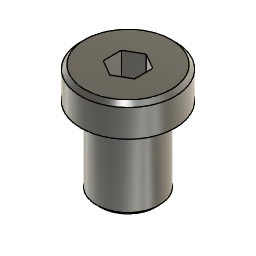
Ensamble+Piezas+SW (Autodesk Fusion 360 archive; units mm, degrees)
design "Cuarta Pieza SW"
Autodesk Fusion 360 part; units mm, degrees
sketch "Sketch1" plane through (0, 0, 0) normal (0, 0, 1) x (1, 0, 0)
  circle A0 centre (0, 0) radius 4
  constraint coincident A0.centre origin
extrude "Extrude1" add sketch "Sketch1" along normal blind 14
sketch "Sketch2" plane through (0, 0, 14) normal (0, 0, 1) x (-1, 0, 0)
  circle A0 centre (0, 0) radius 4
  circle A1 centre (0, 0) radius 6
  constraint coincident A0.centre A1.centre
extrude "Extrude2" add sketch "Sketch2" against normal blind 4
chamfer "Chamfer1" distance 0.5 angle 45 1 edges at (5.594, 2.1697, 14)
chamfer "Chamfer2" distance 0.5 angle 45 1 edges at (-3.7293, -1.4465, 0)
sketch "Sketch3" plane through (0, 0, 14) normal (0, 0, 1) x (-1, 0, 0)
  circle A0 centre (0, 0) radius 5.5
  line L0 (2, -1.1547) -> (2, 1.1547)
  line L1 (-2, 1.1547) -> (-2, -1.1547)
  line L2 (2, -1.1547) -> (0, -2.3094)
  line L3 (0, -2.3094) -> (-2, -1.1547)
  line L4 (2, 1.1547) -> (0, 2.3094)
  line L5 (-2, 1.1547) -> (0, 2.3094)
extrude "Extrude3" cut sketch "Sketch3" against normal blind 4 contours L0 L1 L2 L3 L4 L5
